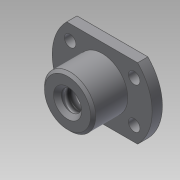
# Autodesk Inventor part: Втулка 12
Saved by Autodesk Inventor 2014 SP1 (Build 180222100, 222)
## iProperties
Created: 2021-12-02
Part Number: Втулка 12
Material: Типовые
Document SubType Name: Modeling
Designer: Украинцев
Mass: 55.5721 g
Surface Area: 145.818 cm^2
Volume: 55.5721 cm^3
Density: 1 g/cm^3
Appearance: По умолчанию
Author: Украинцев
Autodesk Inventor part; units mm, degrees
ref_plane "YZ Plane" through (0, 0, 0) normal (1, 0, 0) x (0, 1, 0)
ref_plane "XZ Plane" through (0, 0, 0) normal (0, 1, 0) x (-1, 0, 0)
ref_plane "XY Plane" through (0, 0, 0) normal (0, 0, 1) x (1, 0, 0)
sketch "Эскиз1" plane through (0, 0, 0) normal (0, 0, 1) x (1, 0, 0)
  line L0 (0, 0) -> (0, 35)
  line L1 (0, 35) -> (39, 35)
  line L2 (39, 35) -> (39, 27)
  line L3 (39, 27) -> (20, 27)
  line L4 (20, 27) -> (20, 0)
  line L5 (20, 0) -> (0, 0)
  dimension "d0" = 78
  dimension "d1" = 40
  dimension "d2" = 8
  dimension "d3" = 35
  constraints: 12 end point, 3 perpendicular, 2 parallel, 1 vertical
  measures "d0" diameter of L2 L0
  measures "d1" diameter of L4 L0
  measures "d2" distance of L1.end L2.end
  measures "d3" distance of L0.start L0.end
revolve "Вращение1" add sketch "Эскиз1" angle 360 about axis through (0, 0, 0) along (0, 1, 0)
sketch "Эскиз2" plane through (0, 35, 0) normal (0, 1, 0) x (1, 0, 0)
  circle A0 centre (0, 0) radius 39 projected
  line L0 (-39, 0) -> (39, 0) construction
  line L1 (-27.6541, 27.5) -> (27.6541, 27.5)
  line L2 (-27.6541, -27.5) -> (27.6541, -27.5)
  line L3 (-25, -16) -> (25, -16) construction
  line L4 (25, -16) -> (25, 16) construction
  line L5 (25, 16) -> (-25, 16) construction
  line L6 (-25, 16) -> (-25, -16) construction
  line L7 (-25, -16) -> (25, 16) construction
  line L8 (25, -16) -> (-25, 16) construction
  circle A1 centre (-25, 16) radius 4.5
  circle A2 centre (-25, -16) radius 4.5
  circle A3 centre (25, -16) radius 4.5
  circle A4 centre (25, 16) radius 4.5
  dimension "d5" = 55
  dimension "d6" = 50
  dimension "d7" = 32
  dimension "d10" = 9
  constraints: 18 end point, 6 point on circle, 5 coincident, 4 centre point, 4 parallel, 3 equal radius, 3 midpoint, 2 horizontal, 1 perpendicular, 1 other
  measures "d5" distance between parallel lines of L2 L1
  measures "d6" distance of L5.end L4.end
  measures "d7" distance of L4.end L3.end
  measures "d10" diameter of A1
extrude "Выдавливание1" cut sketch "Эскиз2" against normal through all contours L1 A0 | A0 L2 | A1 | A2 | A3 | A4
hole "Отверстие1" at (0, 35, 0) direction (0, -1, 0) diameter 16 end through all thread size "TR24x8" class "7H" standard "ISO Metric Trapezoidal Threads"
chamfer "Фаска1" distance 3 angle 45 1 edges at (0, 0, -8)
chamfer "Фаска2" distance 2 angle 45 1 edges at (-20, 0, 0)
